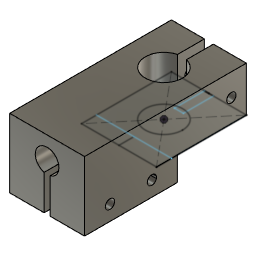
PSB v1 (Autodesk Fusion 360 design; units mm, degrees)
Autodesk Fusion 360 part; units mm, degrees
sketch "Sketch1" plane through (0, 0, 0) normal (0, 0, 1) x (1, 0, 0)
  line L0 (12.5, 15) -> (-12.5, 15)
  line L1 (-12.5, 15) -> (-12.5, -15)
  line L2 (-12.5, -15) -> (12.5, -15)
  line L3 (12.5, -15) -> (12.5, 15)
  line L4 (12.5, 15) -> (-12.5, -15) construction
  line L5 (-12.5, 15) -> (12.5, -15) construction
  circle A0 centre (0, 0) radius 6.2
  line L6 (0, 15) -> (-1.5, 15)
  line L7 (0, 15) -> (-1.5, 15)
  line L8 (0, 15) -> (1.5, 15)
  line L9 (1.5, 5) -> (-1.5, 5)
  line L10 (-1.5, 5) -> (-1.5, 15)
  line L11 (1.5, 5) -> (1.5, 15)
  line L12 (0, -15) -> (0, -10)
  line L13 (0, -10) -> (-12.5, -10)
  line L14 (12.5, -10) -> (0, -10)
  dimension "d1" = 25
  dimension "d2" = 30
  dimension "d3" = 12.4
  constraint horizontal L0
  constraint perpendicular L0 L1
  constraint parallel L0 L2
  constraint parallel L1 L3
  constraint coincident L4 A0.centre
  constraint coincident L5 A0.centre
  constraint coincident A0.centre origin
  constraint midpoint L0 L6.start
  constraint coincident L0 L6.end
  constraint coincident L0 L8.end
  constraint parallel L0 L8
  constraint parallel L8 L9
  constraint perpendicular L7 L10
  constraint perpendicular L8 L11
  constraint midpoint L2 L12.start
  constraint perpendicular L2 L12
  constraint coincident L1 L13.end
  constraint perpendicular L1 L13
  constraint coincident L3 L14.start
  constraint perpendicular L12 L14
  measures "d1" distance of L1.end L2.end
  measures "d2" distance of L0.end L1.end
  measures "d3" diameter of A0
extrude "Extrude1" add sketch "Sketch1" along normal blind 15 contours L0 L1 L3 A0 L10 L11 L13 L14 | L2 L3 L12 L14 | L1 L2 L12 L13
sketch "Sketch2" plane through (0, -15, 0) normal (0, -1, 0) x (1, 0, 0)
  line L0 (-12.5, 0) -> (12.5, 0)
  line L1 (12.5, 0) -> (12.5, 15)
  line L2 (12.5, 15) -> (-12.5, 15)
  line L3 (-12.5, 15) -> (-12.5, 0)
  line L4 (0, 0) -> (0, 7.5)
  circle A0 centre (0, 7.5) radius 3.95
  line L5 (0, 0) -> (1, 0)
  line L6 (0, 0) -> (-1, 0)
  line L7 (-1, 0) -> (-1, 0.2168)
  line L8 (-1, 0.2168) -> (-1, 4.2168)
  line L9 (-1, 4.2168) -> (1, 4.2168)
  line L10 (1, 4.2168) -> (1, 0)
  line L11 (-1, 0) -> (1, 0)
  line L12 (1, 0) -> (1, -8)
  line L13 (1, -8) -> (-1, -8)
  line L14 (-1, -8) -> (-1, 0)
  dimension "d6" = 7.5
  dimension "d7" = 7.9
  dimension "d8" = 4
  constraint coincident L4.start L5.start
  constraint perpendicular L2 L4
  constraint coincident L4.end A0.centre
  constraint coincident L0 L5.end
  constraint coincident L0 L6.end
  constraint perpendicular L6 L7
  constraint perpendicular L6 L8
  constraint perpendicular L4 L9
  constraint perpendicular L0 L10
  constraint horizontal L11
  constraint vertical L12
  constraint horizontal L13
  constraint vertical L14
  measures "d6" distance of L4.start L4.end
  measures "d7" diameter of A0
  measures "d8" distance of L7.end L8.end
extrude "Extrude2" add sketch "Sketch1" against normal blind 8 contours L0 L1 L3 A0 L10 L11 L13 L14 | L2 L3 L12 L14 | L1 L2 L12 L13
extrude "Extrude3" cut sketch "Sketch2" against normal blind 7 contours L0 L4 A0 L6 L7 L8 L11 | L0 L5 L6 L11 L12 L13 L14 | L0 L4 A0 L5 L10 L11 | L4 A0 L8 L9 | L4 A0 L9 L10 | A0 L8 L9 L10
extrude "Extrude4" cut sketch "Sketch1" against normal blind 6 contours L0 L1 L3 A0 L10 L11 L13 L14
sketch "Sketch3" plane through (12.5, 0, 0) normal (1, 0, 0) x (0, 1, 0)
  line L0 (-10, 0) -> (15, 0)
  line L1 (15, 0) -> (15, 15)
  line L2 (15, 15) -> (-15, 15)
  line L3 (-15, 15) -> (-15, -8)
  line L4 (-15, -8) -> (15, -8)
  line L5 (-10, -6) -> (-10, 0)
  line L6 (15, 7.5) -> (10, 7.5)
  circle A0 centre (10, 7.5) radius 1.55
  circle A1 centre (-16.5, -3) radius 1.55
  line L7 (15, -8) -> (15, -6)
  line L8 (15, -6) -> (-10, -6)
  dimension "d15" = 3.1
  dimension "d18" = 3.1
  dimension "d22" = 6.5
  constraint midpoint L1 L6.start
  constraint perpendicular L1 L6
  constraint coincident L6.end A0.centre
  measures "d15" diameter of A0
  measures "d18" diameter of A1
  measures "d22" distance of L5 A1.centre
extrude "Extrude5" cut sketch "Sketch3" against normal blind 25 contours A0
move_face "OffsetFaces1" offset 2 1 faces at (-9.5991, -15, 4.4708)
move_face "OffsetFaces2" offset 2 2 faces at (8.6667, -10, -2) (-4.8333, -10, -2)
move_face "OffsetFaces3" offset 2 1 faces at (-9.5991, -17, 4.4708)
sketch "Sketch4" plane through (0, 0, -8) normal (0, 0, -1) x (1, 0, 0)
  line L0 (1, 19) -> (1, 8)
  line L1 (1, 8) -> (-1, 8)
  line L2 (-1, 8) -> (-1, 19)
  line L3 (-1, 19) -> (-12.5, 19)
  line L4 (-12.5, 19) -> (-12.5, -15)
  line L5 (-12.5, -15) -> (-1.5, -15)
  line L6 (-1.5, -15) -> (-1.5, -6.0158)
  arc A0 (1.5, -6.0158) -> (-1.5, -6.0158) centre (0, 0) ccw
  line L7 (1.5, -6.0158) -> (1.5, -15)
  line L8 (1.5, -15) -> (12.5, -15)
  line L9 (12.5, -15) -> (12.5, 19)
  line L10 (12.5, 19) -> (1, 19)
  line L11 (-1, 8) -> (-12.5, 8)
  line L12 (1, 8) -> (12.5, 8)
  line L13 (1, 8) -> (1, 8)
  line L14 (1, 8) -> (12.5, 8)
  line L15 (-1, 8) -> (-1, 8)
  line L16 (-1, 8) -> (-12.5, 8)
  constraint coincident L1.end L2.start
  constraint coincident L4 L11.end
  constraint perpendicular L4 L11
  constraint coincident L0.end L1.start
  constraint coincident L9 L12.end
  constraint perpendicular L9 L12
  constraint perpendicular L12 L13
  constraint perpendicular L9 L14
  constraint perpendicular L11 L15
  constraint perpendicular L15 L16
extrude "Extrude7" cut sketch "Sketch4" against normal blind 2 contours L1 L4 L5 L6 A0 L7 L8 L9 L11 L12 L14 L16
move_face "OffsetFaces4" offset 5 1 faces at (-9.5991, -19, 4.4708)
extrude "Extrude8" cut sketch "Sketch3" against normal blind 25 contours L3 A1 picked at (-16.7457, -2.5322)
extrude "Extrude9" add 1 faces at (-9.5991, -24, 4.4708) along direction (0, -1, 0) blind 15
sketch "Sketch5" plane through (12.5, 0, 0) normal (1, 0, 0) x (0, 1, 0)
  line L0 (-15, -2.6095) -> (-15, -3.3905)
  arc A0 (-15, -2.6095) -> (-15, -3.3905) centre (-16.5, -3) ccw
  line L1 (-8, -8) -> (-8, 0)
  line L2 (-8, 0) -> (15, 0)
  line L3 (15, 0) -> (15, 15)
  line L4 (15, 15) -> (-39, 15)
  line L5 (-39, 15) -> (-39, -8)
  line L6 (-39, -8) -> (-8, -8)
  circle A1 centre (10, 7.5) radius 1.55
  line L7 (-39, -8) -> (-30.5, -8)
  line L8 (-30.5, -8) -> (-30.5, -3)
  line L9 (-30.5, -3) -> (-39, -3)
  line L10 (-39, -3) -> (-39, -8)
  circle A2 centre (-30.5, -3) radius 1.55
  dimension "d32" = 8.5
  dimension "d33" = 5
  dimension "d34" = 3.1
  constraint horizontal L7
  constraint vertical L8
  constraint horizontal L9
  constraint vertical L10
  constraint coincident L5.end L6.start
  constraint coincident L8.end L9.start
  measures "d32" distance of L5.end L7.end
  measures "d33" distance of L5.end L9.end
  measures "d34" diameter of A2
extrude "Extrude10" cut sketch "Sketch5" against normal blind 25 contours L8 L9 A2 | L8 L9 A2
